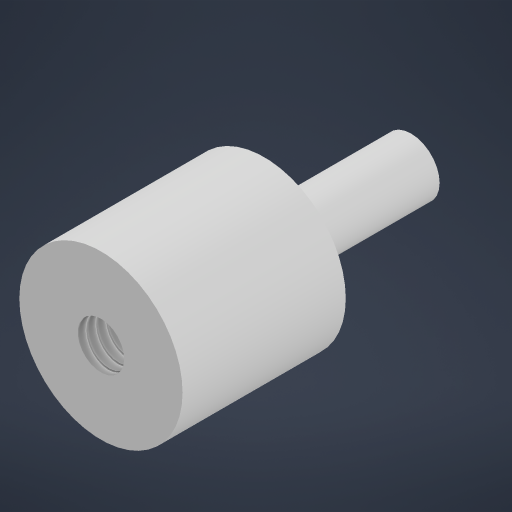
# Autodesk Inventor part: Elbow_Parallel_Rod_V1
Saved by Autodesk Inventor 2024.1 (Build 281209000, 209)
## iProperties
Created: 2023-06-29
Part Number: Elbow_Parallel_Rod_V1
Material: Generic
Document SubType Name: Modeling
Designer: User
Density: 1 g/cm^3
Appearance: Default
Author: User
Autodesk Inventor part; units mm, degrees
ref_plane "YZ Plane" through (0, 0, 0) normal (1, 0, 0) x (0, 1, 0)
ref_plane "XZ Plane" through (0, 0, 0) normal (0, 1, 0) x (-1, 0, 0)
ref_plane "XY Plane" through (0, 0, 0) normal (0, 0, 1) x (1, 0, 0)
sketch "Sketch7" plane through (0, 0, 0) normal (0, 0, 1) x (1, 0, 0)
  circle A0 centre (0, 0) radius 1.75
  dimension "d19" = 3.5
  constraints: 1 centre point, 1 coincident
  measures "d19" diameter of A0
extrude "Extrusion6" add sketch "Sketch7" along normal blind 9
sketch "Sketch8" plane through (0, 0, 9) normal (0, 0, 1) x (1, 0, 0)
  circle A0 centre (0, 0) radius 5
  dimension "d22" = 10
  constraints: 1 centre point, 1 coincident
  measures "d22" diameter of A0
extrude "Extrusion7" add sketch "Sketch8" along normal blind 10
sketch "Sketch9" plane through (0, 0, 19) normal (0, 0, 1) x (1, 0, 0)
  point P0 (0, 0)
  point P1 (0, 0)
  constraints: 1 coincident
hole "Hole1" at (0, 0, 19) direction (0, 0, -1) diameter 2.85 depth 8 thread size "M3.5x0.6" class "6H" standard "ANSI Metric M Profile"
body "Solid2"
